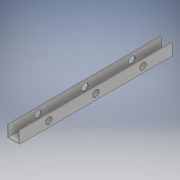
# Autodesk Inventor part: u-channel
Saved by Autodesk Inventor 2018 (Build 220112000, 112)
## iProperties
Created: 2018-06-29
Part Number: u-channel
Material: Generic
Document SubType Name: Modeling
Designer: s-2512711
Density: 1 g/cm^3
Appearance: Default
Author: s-2512711
Autodesk Inventor part; units mm, degrees
ref_plane "YZ Plane" through (0, 0, 0) normal (1, 0, 0) x (0, 1, 0)
ref_plane "XZ Plane" through (0, 0, 0) normal (0, 1, 0) x (-1, 0, 0)
ref_plane "XY Plane" through (0, 0, 0) normal (0, 0, 1) x (1, 0, 0)
sketch "Sketch1" plane through (0, 0, 0) normal (0, 0, 1) x (1, 0, 0)
  line L0 (0, 0) -> (0, 50.8)
  line L1 (0, 50.8) -> (3.175, 50.8)
  line L2 (0, 0) -> (50.8, 0)
  line L3 (50.8, 0) -> (50.8, 50.8)
  line L4 (50.8, 50.8) -> (47.625, 50.8)
  line L5 (50.8, 0) -> (50.8, 3.175)
  line L6 (47.625, 3.175) -> (3.175, 3.175)
  line L7 (3.175, 3.175) -> (3.175, 50.8)
  line L8 (47.625, 50.8) -> (47.625, 3.175)
  dimension "d0" = 50.8
  dimension "d1" = 3.175
  dimension "d2" = 50.8
  dimension "d3" = 3.175
  dimension "d4" = 50.8
  dimension "d5" = 3.175
  constraints: 18 end point, 6 perpendicular, 1 horizontal, 1 point on line, 1 vertical
  measures "d0" distance of L0.start L0.end
  measures "d1" distance of L0.end L1.end
  measures "d2" distance of L0.start L2.end
  measures "d3" distance of L3.end L4.end
  measures "d4" distance of L2.end L3.end
  measures "d5" distance of L2.end L5.end
extrude "Extrusion1" add sketch "Sketch1" along normal blind 660.4
sketch "Sketch2" plane through (50.8, 0, 0) normal (1, 0, 0) x (0, 0, -1)
  line L0 (0, 50.8) -> (-660.4, 50.8) projected
  line L1 (-330.2, 50.8) -> (-330.2, 0)
  line L2 (0, 0) -> (-660.4, 0) projected
  line L3 (0, 50.8) -> (0, 3.175) projected
  line L4 (0, 50.8) -> (-127, 50.8)
  line L5 (-127, 50.8) -> (-127, 0)
  line L6 (-660.4, 50.8) -> (-533.4, 50.8)
  line L7 (-533.4, 50.8) -> (-533.4, 0)
  circle A0 centre (-330.2, 25.4) radius 14.2875
  circle A1 centre (-533.4, 25.4) radius 14.2875
  circle A2 centre (-127, 25.4) radius 14.2875
  dimension "d8" = 127
  dimension "d9" = 127
  dimension "d10" = 28.575
  constraints: 10 end point, 5 midpoint, 3 centre point, 2 perpendicular, 2 point on line, 1 horizontal
  measures "d8" distance of L0.start L4.end
  measures "d9" distance of L0.end L6.end
  measures "d10" diameter of A0
extrude "Extrusion2" cut sketch "Sketch2" against normal blind 53.975 contours A2 L5 | L5 A2 | A0 L1 | L1 A0 | A1 L7 | L7 A1
body "Solid1"
